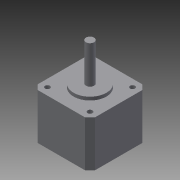
# Autodesk Inventor part: NEMA17
Saved by Autodesk Inventor 2013 SP2 (Build 170200200, 200)
## iProperties
Created: 2017-01-25
Part Number: NEMA17
Material: Generic
Document SubType Name: Modeling
Designer: Herman de Vries
Density: 1 g/cm^3
Author: Herman de Vries
Autodesk Inventor part; units mm, degrees
ref_plane "YZ Plane" through (0, 0, 0) normal (1, 0, 0) x (0, 1, 0)
ref_plane "XZ Plane" through (0, 0, 0) normal (0, 1, 0) x (-1, 0, 0)
ref_plane "XY Plane" through (0, 0, 0) normal (0, 0, 1) x (1, 0, 0)
sketch "Sketch1" plane through (0, 0, 0) normal (0, 0, 1) x (1, 0, 0)
  line L0 (0, 0) -> (35, 0)
  line L1 (35, 0) -> (35, 35)
  line L2 (35, 35) -> (0, 35)
  line L3 (0, 35) -> (0, 0)
  line L4 (4.5, 30.5) -> (30.5, 30.5) construction
  line L5 (30.5, 30.5) -> (30.5, 4.5) construction
  line L6 (30.5, 4.5) -> (4.5, 4.5) construction
  line L7 (4.5, 4.5) -> (4.5, 30.5) construction
  circle A0 centre (4.5, 30.5) radius 1.5
  circle A1 centre (30.5, 30.5) radius 1.5
  circle A2 centre (30.5, 4.5) radius 1.5
  circle A3 centre (4.5, 4.5) radius 1.5
  circle A4 centre (17.5, 17.5) radius 2.5
  point P0 (17.5, 35)
  point P1 (35, 17.5)
  dimension "d0" = 35
  dimension "d1" = 35
  dimension "d2" = 26
  dimension "d3" = 3
  dimension "d4" = 3
  dimension "d5" = 3
  dimension "d6" = 3
  dimension "d9" = 5
  constraints: 16 end point, 5 centre point, 4 coincident, 4 parallel, 2 midpoint, 2 perpendicular, 1 horizontal, 1 horizontal alignment, 1 vertical alignment, 3 other
  measures "d0" distance of L2.end L1.end
  measures "d1" distance of L1.end L0.end
  measures "d2" distance of L4.start L4.end
  measures "d3" diameter of A0
  measures "d4" diameter of A1
  measures "d5" diameter of A2
  measures "d6" diameter of A3
  measures "d9" diameter of A4
extrude "Extrusion1" add sketch "Sketch1" along normal blind 28
chamfer "Chamfer1" distance 3 angle 45 4 edges at (35, 35, 14) (35, 0, 14) (0, 0, 14) (0, 35, 14)
sketch "Sketch2" plane through (0, 0, 28) normal (0, 0, 1) x (1, 0, 0)
  circle A0 centre (17.5, 17.5) radius 2.5 construction
  circle A1 centre (17.5, 17.5) radius 10
  point P0 (0, 0)
  dimension "d13" = 20
  constraints: 1 centre point, 1 coincident
  measures "d13" diameter of A1
sketch "Sketch3" plane through (0, 0, 28) normal (0, 0, 1) x (1, 0, 0)
  circle A0 centre (17.5, 17.5) radius 2.5 projected
  point P0 (0, 0)
extrude "Extrusion2" add sketch "Sketch3" along normal blind 25
extrude "Extrusion3" add sketch "Sketch2" along normal blind 2
body "Solid1"
